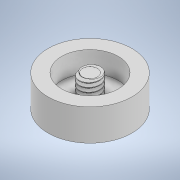
# Autodesk Inventor part: piston clamp adapter with threads
Saved by Autodesk Inventor 2020 (Build 240168000, 168)
## iProperties
Created: 2024-01-11
Part Number: piston clamp adapter with threads
Material: Generic
Document SubType Name: Modeling
Designer: Beaucage
Density: 1 g/cm^3
Appearance: Default
Author: Beaucage
Autodesk Inventor part; units mm, degrees
ref_plane "YZ Plane" through (0, 0, 0) normal (1, 0, 0) x (0, 1, 0)
ref_plane "XZ Plane" through (0, 0, 0) normal (0, 1, 0) x (-1, 0, 0)
ref_plane "XY Plane" through (0, 0, 0) normal (0, 0, 1) x (1, 0, 0)
sketch "Sketch1" plane through (0, 0, 0) normal (0, 1, 0) x (-1, 0, 0)
  circle A0 centre (0, 0) radius 12.7
  dimension "d0" = 25.4
  constraints: 1 centre point, 1 coincident
  measures "d0" diameter of A0
extrude "Extrusion1" add sketch "Sketch1" along normal blind 9.525
sketch "Sketch2" plane through (0, 9.525, 0) normal (0, 1, 0) x (1, 0, 0)
  circle A0 centre (0, 0) radius 8.5725
  dimension "d3" = 17.145
  constraints: 1 centre point, 1 coincident
  measures "d3" diameter of A0
extrude "Extrusion2" cut sketch "Sketch2" against normal blind 6.35
sketch "Sketch3" plane through (0, 3.175, 0) normal (0, 1, 0) x (1, 0, 0)
  circle A0 centre (0, 0) radius 3.175
  dimension "d6" = 6.35
  constraints: 1 centre point, 1 coincident
  measures "d6" diameter of A0
extrude "Extrusion3" add sketch "Sketch3" along normal blind 6.35
thread "Thread1" size "1/4-20 UNC" class "2A" standard "ANSI Unified Screw Threads" length 6.35
sketch "Sketch8" plane through (0, 9.525, 0) normal (1, 0, 0) x (0, 0, 1)
  line L0 (3.175, 0) -> (3.175, 6.35)
  line L1 (3.175, 6.35) -> (2.2333, 6.35)
  line L2 (2.2333, 6.35) -> (2.2333, 0)
  line L3 (2.2333, 0) -> (3.175, 0)
  line L4 (0, -3.5669) -> (0, 11.707) projected
  constraints: 8 end point
revolve "Revolution3" cut sketch "Sketch8" angle 360 about axis through (0, 9.525, 0) along (0, -1, 0)
sketch "Sketch9" plane through (0, 9.525, 0) normal (1, 0, 0) x (0, 0, 1)
  line L0 (3.175, 0) -> (3.175, 6.35)
  line L1 (3.175, 6.35) -> (2.2333, 6.35)
  line L2 (2.2333, 6.35) -> (2.2333, 0)
  line L3 (2.2333, 0) -> (3.175, 0)
  line L4 (0, -3.5669) -> (0, 11.707) projected
  constraints: 8 end point
revolve "Revolution4" add sketch "Sketch9" angle 360 about axis through (0, 9.525, 0) along (0, -1, 0) separate body
sketch "Sketch7" plane through (0, 9.525, 0) normal (-1, 0, 0) x (0, -1, 0)
  line L0 (-0.7409, -2.2977) -> (-0.6351, -2.2977) construction
  line L1 (0.1057, -3.1109) -> (-0.0001, -3.3143) construction
  line L2 (-1.2701, -3.3143) -> (-1.3759, -3.1109) construction
  line L3 (-0.5293, -2.2977) -> (-0.6351, -2.0944) construction
  line L4 (-0.6351, -2.0944) -> (-0.7409, -2.2977) construction
  line L5 (-1.2701, -3.3143) -> (-1.1643, -3.1109) construction
  line L6 (-0.5293, -2.2977) -> (-0.1059, -3.1109)
  line L7 (-1.3759, -3.1109) -> (-1.1643, -3.1109) construction
  arc A0 (-1.3759, -3.1109) -> (-1.2701, -3.1752) centre (-1.2701, -3.0559) ccw construction
  line L8 (0.1057, -3.1109) -> (-0.1059, -3.1109) construction
  line L9 (-1.2701, -3.3143) -> (-1.2701, -3.1109) construction
  line L10 (-0.0001, -3.3143) -> (-0.0001, -3.1109) construction
  line L11 (-0.6351, -2.0944) -> (-0.6351, -2.2335) construction
  line L12 (-1.2701, -3.1752) -> (-0.0001, -3.1752)
  arc A1 (-1.2701, -3.1752) -> (-1.1643, -3.1109) centre (-1.2701, -3.0559) ccw
  line L13 (-0.1059, -3.1109) -> (-0.0001, -3.3143) construction
  line L14 (-1.1643, -3.1109) -> (-0.7409, -2.2977)
  line L15 (-0.0001, -0.0002) -> (-0.0001, 0.0177)
  line L16 (-0.0001, 0.0177) -> (-0.0001, -0.0002)
  line L17 (-0.0001, -0.0002) -> (0.0334, -0.0002)
  arc A2 (-0.1059, -3.1109) -> (-0.0001, -3.1752) centre (-0.0001, -3.0559) ccw
  arc A3 (-0.0001, -3.1752) -> (0.1057, -3.1109) centre (-0.0001, -3.0559) ccw construction
  arc A4 (-0.6351, -2.2335) -> (-0.7409, -2.2977) centre (-0.6351, -2.3528) ccw
  arc A5 (-0.5293, -2.2977) -> (-0.6351, -2.2335) centre (-0.6351, -2.3528) ccw
  line L18 (-0.6351, -2.2335) -> (-0.6351, -2.2977) construction
  line L19 (-0.6351, -2.2977) -> (-0.5293, -2.2977) construction
  dimension "d30" = 55
  dimension "d31" = 0.2033
  dimension "d32" = 0.2033
  dimension "Sketch7_ThreadOffset" = 0
  dimension "Sketch7_MajorRadius" = 3.175
  dimension "d35" = 1.27
  dimension "Sketch7_MinorRadius" = 2.2333
  constraints: 40 end point, 12 point on circle, 10 parallel, 8 tangent, 6 centre point, 6 collinear, 2 midpoint, 2 point on line, 1 horizontal, 1 perpendicular, 3 other
  measures "d30" angle of L6 L14
  measures "d31" distance of L3.end L0.end
  measures "d32" distance of L1.end L10.end
  measures "Sketch7_ThreadOffset" distance between parallel lines of L15 L10
  measures "Sketch7_MajorRadius" distance from line of L12 L15.start
  measures "d35" distance from line of L1.end L9
  measures "Sketch7_MinorRadius" distance edge to line of A5 L17
coil "Coil2" sketch "Sketch7" operation cut axis through (0, 9.525, 0) along (0, -1, 0) pitch 1.2713 turns 6.993007 hand right bodies 2
equation "\"d30\" = d37"
equation "\"d31\" = 0.160083 * Sketch7_Pitch"
equation "\"d32\" = 0.160083 * Sketch7_Pitch"
equation "\"d35\" = Sketch7_Pitch"
equation "\"d18\" = 55deg"
equation "\"Sketch4_Pitch\" = 1.27"
equation "\"d37\" = 55deg"
equation "\"Sketch7_Pitch\" = 1.27"
body "Solid1"
body "Solid3"
